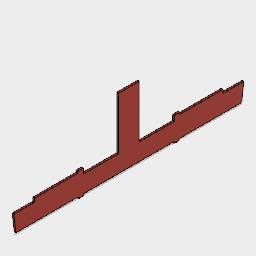
鳥居 (Autodesk Fusion 360 archive; units mm, degrees)
design "貫"
Autodesk Fusion 360 part; units mm, degrees
sketch "Sketch1" plane through (0, 0, 0) normal (1, 0, 0) x (0, 0, -1)
  line L0 (-170.107, 63.9648) -> (159.3036, 63.9648)
  line L1 (159.3036, 63.9648) -> (159.3036, 38.9648)
  line L2 (159.3036, 38.9648) -> (-170.107, 38.9648)
  line L3 (-170.107, 38.9648) -> (-170.107, 63.9648)
  line L4 (-5.4017, 63.9648) -> (-5.4017, 38.9648) construction
  line L5 (94.5983, 63.9648) -> (94.5983, 38.9648) construction
  line L6 (59.5983, 63.9648) -> (129.5983, 63.9648)
  line L7 (129.5983, 63.9648) -> (129.5983, 68.9648)
  line L8 (129.5983, 68.9648) -> (59.5983, 68.9648)
  line L9 (59.5983, 68.9648) -> (59.5983, 63.9648)
  line L10 (-70.4017, 68.9648) -> (-70.4017, 63.9648)
  line L11 (-140.4017, 68.9648) -> (-70.4017, 68.9648)
  line L12 (-140.4017, 63.9648) -> (-140.4017, 68.9648)
  line L13 (159.3036, 63.9648) -> (156.3036, 38.9648)
  line L14 (-170.107, 63.9648) -> (-167.107, 38.9648)
  line L15 (-20.4017, 63.9648) -> (9.5983, 63.9648)
  line L16 (9.5983, 63.9648) -> (9.5983, 138.9648)
  line L17 (9.5983, 138.9648) -> (-20.4017, 138.9648)
  line L18 (-20.4017, 138.9648) -> (-20.4017, 63.9648)
  line L19 (-20.4017, 138.9648) -> (-10.4017, 138.9648)
  line L20 (9.5983, 138.9648) -> (-0.0785, 138.9648)
  line L21 (-78.4017, 68.9648) -> (67.5983, 68.9648) construction
  line L22 (-77.4017, 38.9648) -> (66.5983, 38.9648) construction
  line L23 (-78.485, 71.4648) -> (-77.3184, 36.4648)
  line L24 (-78.485, 71.4648) -> (-70.4017, 71.4648)
  line L25 (-70.4017, 71.4648) -> (-70.4017, 68.9648)
  line L26 (-77.3184, 36.4648) -> (-70.4017, 36.4648)
  line L27 (-70.4017, 36.4648) -> (-70.4017, 38.9648)
  line L28 (67.6816, 71.4648) -> (66.515, 36.4648)
  line L29 (67.6816, 71.4648) -> (59.5983, 71.4648)
  line L30 (59.5983, 71.4648) -> (59.5983, 68.9648)
  line L31 (66.515, 36.4648) -> (59.5983, 36.4648)
  line L32 (59.5983, 36.4648) -> (59.5983, 38.9648)
  point P0 (-5.4017, 68.9648)
  point P1 (-5.4017, 63.9648)
  point P2 (-5.4017, 38.9648)
  dimension "d4" = 100
  dimension "d5" = 30
  dimension "d6" = 70
  dimension "d7" = 3
  dimension "d12" = 75
  dimension "d14" = 30
  dimension "d17" = 10
  dimension "d21" = 5
  dimension "d22" = 146
  dimension "d24" = 144
  dimension "d25" = 2.5
  measures "d4" distance of P1 L5.start
  measures "d5" distance of L2 L8
  measures "d6" distance of L7.end L8.end
  measures "d7" distance of L1.end L13.end
  measures "d12" distance of L15.start L17.end
  measures "d14" distance of L16.end L17.end
  measures "d17" distance of L17.end L19.end
  measures "d21" distance of L0 L11
  measures "d22" distance of L21.start L21.end
  measures "d24" distance of L22.start L22.end
  measures "d25" distance of L10.start L24.end
extrude "Extrude1" add sketch "Sketch1" along normal blind 2.5 contours L0 L2 L14 L23 | L0 L11 L12 L23 | L0 L10 L11 L23 | L0 L2 L6 L15 L23 L28 | L2 L23 L26 L27 | L11 L23 L24 L25 | L0 L15 L16 L17 L18 L19 L20 | L2 L28 L31 L32 | L0 L2 L6 L13 L28 | L0 L6 L8 L9 L28 | L0 L6 L7 L8 L28 | L8 L28 L29 L30
equation "nuki_height = 30 mm"
equation "leg_distance = 200 mm"
equation "d4 = leg_distance / 2"
equation "d5 = nuki_height"
equation "d8 = thickness"
equation "thickness = 2.5 mm"
equation "i = 60 mm"
equation "d12 = i + 15 mm"
equation "j = 30 mm"
equation "d14 = j"
equation "d17 = d14 / 3"
